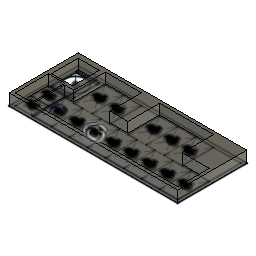
keyboard setup v5 (Autodesk Fusion 360 design; units mm, degrees)
Autodesk Fusion 360 part; units mm, degrees
sketch "Sketch1" plane through (0, 0, 0) normal (0, 0, 1) x (1, 0, 0)
  circle A0 centre (0, 0) radius 2
  line L0 (0, 0) -> (5.08, 0) construction
  circle A1 centre (5.08, 0) radius 0.85
  line L1 (0, 0) -> (2.54, 0) construction
  line L2 (2.54, 0) -> (2.54, 5.08) construction
  line L3 (2.54, 5.08) -> (0, 5.08) construction
  line L4 (0, 5.08) -> (0, 0) construction
  circle A2 centre (2.54, 5.08) radius 1.25
  line L5 (0, 0) -> (-3.81, 0) construction
  line L6 (-3.81, 0) -> (-3.81, 2.54) construction
  line L7 (-3.81, 2.54) -> (0, 2.54) construction
  line L8 (0, 2.54) -> (0, 0) construction
  circle A3 centre (-3.81, 2.54) radius 1.25
  circle A4 centre (-5.08, 0) radius 0.85
  line L9 (12, 21) -> (-12, 21)
  line L10 (-12, 21) -> (-12, -21)
  line L11 (-12, -21) -> (12, -21)
  line L12 (12, -21) -> (12, 21) construction
  line L13 (12, 21) -> (-12, -21) construction
  line L14 (-12, 21) -> (12, -21) construction
  line L15 (12, 21) -> (12, -21) construction
  line L16 (36, 21) -> (12, 21) construction
  line L17 (12, -21) -> (36, -21)
  line L18 (26.54, 5.08) -> (24, 5.08) construction
  line L19 (36, 21) -> (12, -21) construction
  line L20 (12, 21) -> (36, -21) construction
  circle A5 centre (24, 0) radius 2
  line L21 (36, -21) -> (36, 21) construction
  line L22 (24, 5.08) -> (24, 0) construction
  line L23 (24, 0) -> (29.08, 0) construction
  circle A6 centre (20.19, 2.54) radius 1.25
  line L24 (24, 2.54) -> (24, 0) construction
  line L25 (24, 0) -> (26.54, 0) construction
  circle A7 centre (18.92, 0) radius 0.85
  circle A8 centre (29.08, 0) radius 0.85
  line L26 (24, 0) -> (20.19, 0) construction
  line L27 (26.54, 0) -> (26.54, 5.08) construction
  circle A9 centre (26.54, 5.08) radius 1.25
  line L28 (20.19, 0) -> (20.19, 2.54) construction
  line L29 (20.19, 2.54) -> (24, 2.54) construction
  line L30 (36, 21) -> (36, -21) construction
  line L31 (60, 21) -> (36, 21)
  line L32 (36, -21) -> (60, -21)
  line L33 (50.54, 5.08) -> (48, 5.08) construction
  line L34 (60, 21) -> (36, -21) construction
  line L35 (36, 21) -> (60, -21) construction
  circle A10 centre (48, 0) radius 2
  line L36 (60, -21) -> (60, 21) construction
  line L37 (48, 5.08) -> (48, 0) construction
  line L38 (48, 0) -> (53.08, 0) construction
  circle A11 centre (44.19, 2.54) radius 1.25
  line L39 (48, 2.54) -> (48, 0) construction
  line L40 (48, 0) -> (50.54, 0) construction
  circle A12 centre (42.92, 0) radius 0.85
  circle A13 centre (53.08, 0) radius 0.85
  line L41 (48, 0) -> (44.19, 0) construction
  line L42 (50.54, 0) -> (50.54, 5.08) construction
  circle A14 centre (50.54, 5.08) radius 1.25
  line L43 (44.19, 0) -> (44.19, 2.54) construction
  line L44 (44.19, 2.54) -> (48, 2.54) construction
  line L45 (60, 21) -> (60, -21) construction
  line L46 (84, 21) -> (60, 21)
  line L47 (60, -21) -> (84, -21)
  line L48 (74.54, 5.08) -> (72, 5.08) construction
  line L49 (84, 21) -> (60, -21) construction
  line L50 (60, 21) -> (84, -21) construction
  circle A15 centre (72, 0) radius 2
  line L51 (84, -21) -> (84, 21) construction
  line L52 (72, 5.08) -> (72, 0) construction
  line L53 (72, 0) -> (77.08, 0) construction
  circle A16 centre (68.19, 2.54) radius 1.25
  line L54 (72, 2.54) -> (72, 0) construction
  line L55 (72, 0) -> (74.54, 0) construction
  circle A17 centre (66.92, 0) radius 0.85
  circle A18 centre (77.08, 0) radius 0.85
  line L56 (72, 0) -> (68.19, 0) construction
  line L57 (74.54, 0) -> (74.54, 5.08) construction
  circle A19 centre (74.54, 5.08) radius 1.25
  line L58 (68.19, 0) -> (68.19, 2.54) construction
  line L59 (68.19, 2.54) -> (72, 2.54) construction
  line L60 (84, 21) -> (84, -21) construction
  line L61 (108, 21) -> (84, 21) construction
  line L62 (84, -21) -> (108, -21)
  line L63 (98.54, 5.08) -> (96, 5.08) construction
  line L64 (108, 21) -> (84, -21) construction
  line L65 (84, 21) -> (108, -21) construction
  circle A20 centre (96, 0) radius 2
  line L66 (108, -21) -> (108, 21) construction
  line L67 (96, 5.08) -> (96, 0) construction
  line L68 (96, 0) -> (101.08, 0) construction
  circle A21 centre (92.19, 2.54) radius 1.25
  line L69 (96, 2.54) -> (96, 0) construction
  line L70 (96, 0) -> (98.54, 0) construction
  circle A22 centre (90.92, 0) radius 0.85
  circle A23 centre (101.08, 0) radius 0.85
  line L71 (96, 0) -> (92.19, 0) construction
  line L72 (98.54, 0) -> (98.54, 5.08) construction
  circle A24 centre (98.54, 5.08) radius 1.25
  line L73 (92.19, 0) -> (92.19, 2.54) construction
  line L74 (92.19, 2.54) -> (96, 2.54) construction
  line L75 (108, 21) -> (108, -21) construction
  line L76 (132, 21) -> (108, 21) construction
  line L77 (108, -21) -> (132, -21)
  line L78 (122.54, 5.08) -> (120, 5.08) construction
  line L79 (132, 21) -> (108, -21) construction
  line L80 (108, 21) -> (132, -21) construction
  circle A25 centre (120, 0) radius 2
  line L81 (132, -21) -> (132, 21) construction
  line L82 (120, 5.08) -> (120, 0) construction
  line L83 (120, 0) -> (125.08, 0) construction
  circle A26 centre (116.19, 2.54) radius 1.25
  line L84 (120, 2.54) -> (120, 0) construction
  line L85 (120, 0) -> (122.54, 0) construction
  circle A27 centre (114.92, 0) radius 0.85
  circle A28 centre (125.08, 0) radius 0.85
  line L86 (120, 0) -> (116.19, 0) construction
  line L87 (122.54, 0) -> (122.54, 5.08) construction
  circle A29 centre (122.54, 5.08) radius 1.25
  line L88 (116.19, 0) -> (116.19, 2.54) construction
  line L89 (116.19, 2.54) -> (120, 2.54) construction
  line L90 (132, 21) -> (132, -21) construction
  line L91 (156, 21) -> (132, 21)
  line L92 (132, -21) -> (156, -21)
  line L93 (146.54, 5.08) -> (144, 5.08) construction
  line L94 (156, 21) -> (132, -21) construction
  line L95 (132, 21) -> (156, -21) construction
  circle A30 centre (144, 0) radius 2
  line L96 (156, -21) -> (156, 21) construction
  line L97 (144, 5.08) -> (144, 0) construction
  line L98 (144, 0) -> (149.08, 0) construction
  circle A31 centre (140.19, 2.54) radius 1.25
  line L99 (144, 2.54) -> (144, 0) construction
  line L100 (144, 0) -> (146.54, 0) construction
  circle A32 centre (138.92, 0) radius 0.85
  circle A33 centre (149.08, 0) radius 0.85
  line L101 (144, 0) -> (140.19, 0) construction
  line L102 (146.54, 0) -> (146.54, 5.08) construction
  circle A34 centre (146.54, 5.08) radius 1.25
  line L103 (140.19, 0) -> (140.19, 2.54) construction
  line L104 (140.19, 2.54) -> (144, 2.54) construction
  line L105 (156, 21) -> (156, -21) construction
  line L106 (180, 21) -> (156, 21)
  line L107 (156, -21) -> (180, -21)
  line L108 (170.54, 5.08) -> (168, 5.08) construction
  line L109 (180, 21) -> (156, -21) construction
  line L110 (156, 21) -> (180, -21) construction
  circle A35 centre (168, 0) radius 2
  line L111 (180, -21) -> (180, 21)
  line L112 (168, 5.08) -> (168, 0) construction
  line L113 (168, 0) -> (173.08, 0) construction
  circle A36 centre (164.19, 2.54) radius 1.25
  line L114 (168, 2.54) -> (168, 0) construction
  line L115 (168, 0) -> (170.54, 0) construction
  circle A37 centre (162.92, 0) radius 0.85
  circle A38 centre (173.08, 0) radius 0.85
  line L116 (168, 0) -> (164.19, 0) construction
  line L117 (170.54, 0) -> (170.54, 5.08) construction
  circle A39 centre (170.54, 5.08) radius 1.25
  line L118 (164.19, 0) -> (164.19, 2.54) construction
  line L119 (164.19, 2.54) -> (168, 2.54) construction
  line L120 (48, 0) -> (53.08, 0) construction
  circle A40 centre (48, 0) radius 2
  line L121 (50.54, 5.08) -> (48, 5.08) construction
  circle A41 centre (42.92, 0) radius 0.85
  line L122 (48, 0) -> (44.19, 0) construction
  line L123 (44.19, 2.54) -> (48, 2.54) construction
  circle A42 centre (50.54, 5.08) radius 0.75
  circle A43 centre (53.08, 0) radius 0.85
  line L124 (50.54, 0) -> (50.54, 5.08) construction
  circle A44 centre (44.19, 2.54) radius 0.75
  line L125 (48, 5.08) -> (48, 0) construction
  line L126 (44.19, 0) -> (44.19, 2.54) construction
  line L127 (48, 2.54) -> (48, 0) construction
  line L128 (48, 0) -> (50.54, 0) construction
  line L129 (8.19, 44.54) -> (12, 44.54) construction
  circle A45 centre (6.92, 42) radius 0.85
  line L130 (12, 42) -> (8.19, 42) construction
  line L131 (12, 44.54) -> (12, 42) construction
  circle A46 centre (17.08, 42) radius 0.85
  line L132 (14.54, 42) -> (14.54, 47.08) construction
  circle A47 centre (12, 42) radius 2
  line L133 (14.54, 47.08) -> (12, 47.08) construction
  circle A48 centre (14.54, 47.08) radius 1.25
  circle A49 centre (8.19, 44.54) radius 1.25
  line L134 (12, 42) -> (14.54, 42) construction
  line L135 (12, 42) -> (17.08, 42) construction
  line L136 (12, 47.08) -> (12, 42) construction
  line L137 (8.19, 42) -> (8.19, 44.54) construction
  line L138 (24, 63) -> (0, 63) construction
  line L139 (0, 63) -> (0, 21)
  line L140 (0, 21) -> (24, 21) construction
  line L141 (24, 21) -> (24, 63) construction
  line L142 (24, 63) -> (0, 21) construction
  line L143 (0, 63) -> (24, 21) construction
  circle A50 centre (36, 42) radius 2
  line L144 (32.19, 44.54) -> (36, 44.54) construction
  line L145 (36, 42) -> (41.08, 42) construction
  line L146 (48, 63) -> (24, 63) construction
  circle A51 centre (38.54, 47.08) radius 1.25
  line L147 (24, 63) -> (24, 21) construction
  line L148 (24, 21) -> (48, 21) construction
  line L149 (48, 63) -> (24, 21) construction
  circle A52 centre (30.92, 42) radius 0.85
  line L150 (36, 47.08) -> (36, 42) construction
  line L151 (36, 42) -> (32.19, 42) construction
  line L152 (36, 42) -> (38.54, 42) construction
  line L153 (36, 44.54) -> (36, 42) construction
  circle A53 centre (41.08, 42) radius 0.85
  line L154 (32.19, 42) -> (32.19, 44.54) construction
  circle A54 centre (32.19, 44.54) radius 1.25
  line L155 (38.54, 47.08) -> (36, 47.08) construction
  line L156 (38.54, 42) -> (38.54, 47.08) construction
  line L157 (24, 63) -> (48, 21) construction
  line L158 (48, 21) -> (48, 63)
  line L159 (96, 63) -> (72, 63) construction
  line L160 (84, 44.54) -> (84, 42) construction
  circle A55 centre (102.92, 42) radius 0.85
  line L161 (108, 42) -> (104.19, 42) construction
  line L162 (104.19, 42) -> (104.19, 44.54) construction
  circle A56 centre (86.54, 47.08) radius 1.25
  line L163 (84, 42) -> (86.54, 42) construction
  line L164 (84, 47.08) -> (84, 42) construction
  circle A57 centre (110.54, 47.08) radius 1.25
  circle A58 centre (80.19, 44.54) radius 1.25
  line L165 (84, 42) -> (80.19, 42) construction
  line L166 (108, 47.08) -> (108, 42) construction
  line L167 (96, 21) -> (96, 63) construction
  line L168 (120, 63) -> (96, 21) construction
  circle A59 centre (113.08, 42) radius 0.85
  circle A60 centre (108, 42) radius 2
  line L169 (120, 63) -> (96, 63) construction
  line L170 (110.54, 47.08) -> (108, 47.08) construction
  line L171 (86.54, 47.08) -> (84, 47.08) construction
  line L172 (96, 21) -> (120, 21) construction
  line L173 (86.54, 42) -> (86.54, 47.08) construction
  line L174 (96, 63) -> (120, 21) construction
  line L175 (108, 44.54) -> (108, 42) construction
  circle A61 centre (84, 42) radius 2
  circle A62 centre (78.92, 42) radius 0.85
  line L176 (108, 42) -> (110.54, 42) construction
  line L177 (80.19, 44.54) -> (84, 44.54) construction
  line L178 (72, 21) -> (96, 21) construction
  line L179 (104.19, 44.54) -> (108, 44.54) construction
  circle A63 centre (104.19, 44.54) radius 1.25
  line L180 (120, 21) -> (120, 63) construction
  line L181 (80.19, 42) -> (80.19, 44.54) construction
  line L182 (72, 63) -> (96, 21) construction
  line L183 (84, 42) -> (89.08, 42) construction
  line L184 (110.54, 42) -> (110.54, 47.08) construction
  line L185 (96, 63) -> (72, 21) construction
  circle A64 centre (89.08, 42) radius 0.85
  line L186 (108, 42) -> (113.08, 42) construction
  line L187 (72, 63) -> (72, 21)
  line L188 (96, 63) -> (96, 21) construction
  circle A65 centre (132, 42) radius 2
  line L189 (128.19, 44.54) -> (132, 44.54) construction
  line L190 (132, 42) -> (137.08, 42) construction
  line L191 (144, 63) -> (120, 63) construction
  circle A66 centre (134.54, 47.08) radius 1.25
  line L192 (120, 63) -> (120, 21) construction
  line L193 (120, 21) -> (144, 21) construction
  line L194 (144, 63) -> (120, 21) construction
  circle A67 centre (126.92, 42) radius 0.85
  line L195 (132, 47.08) -> (132, 42) construction
  line L196 (132, 42) -> (128.19, 42) construction
  line L197 (132, 42) -> (134.54, 42) construction
  line L198 (132, 44.54) -> (132, 42) construction
  circle A68 centre (137.08, 42) radius 0.85
  line L199 (128.19, 42) -> (128.19, 44.54) construction
  circle A69 centre (128.19, 44.54) radius 1.25
  line L200 (134.54, 47.08) -> (132, 47.08) construction
  line L201 (134.54, 42) -> (134.54, 47.08) construction
  line L202 (120, 63) -> (144, 21) construction
  line L203 (144, 21) -> (144, 63)
  line L204 (-12, -21) -> (180, -21)
  line L205 (180, -21) -> (180, 63)
  line L206 (180, 63) -> (-12, 63)
  line L207 (-12, 63) -> (-12, -21)
  circle A70 centre (-25, -10) radius 2
  line L208 (-25, -7.46) -> (-25, -10) construction
  circle A71 centre (-22.46, -4.92) radius 1.25
  line L209 (-25, -4.92) -> (-25, -10) construction
  circle A72 centre (-30.08, -10) radius 0.85
  line L210 (-28.81, -7.46) -> (-25, -7.46) construction
  line L211 (-25, -10) -> (-22.46, -10) construction
  circle A73 centre (-19.92, -10) radius 0.85
  line L212 (-25, -10) -> (-28.81, -10) construction
  line L213 (-22.46, -10) -> (-22.46, -4.92) construction
  line L214 (-22.46, -4.92) -> (-25, -4.92) construction
  circle A74 centre (-28.81, -7.46) radius 1.25
  line L215 (-28.81, -10) -> (-28.81, -7.46) construction
  line L216 (-25, -10) -> (-19.92, -10) construction
  line L217 (-14, 1) -> (-36, 1)
  line L218 (-36, 1) -> (-36, -21)
  line L219 (-36, -21) -> (-14, -21)
  line L220 (-14, -21) -> (-14, 1)
  line L221 (-14, 1) -> (-36, -21) construction
  line L222 (-36, 1) -> (-14, -21) construction
  line L223 (-36, 23) -> (-14, 1) construction
  line L224 (-25, 12) -> (-22.46, 12) construction
  line L225 (-28.81, 12) -> (-28.81, 14.54) construction
  line L226 (-28.81, 14.54) -> (-25, 14.54) construction
  line L227 (-36, 23) -> (-36, 1)
  line L228 (-36, 1) -> (-14, 1)
  line L229 (-25, 12) -> (-19.92, 12) construction
  line L230 (-25, 14.54) -> (-25, 12) construction
  circle A75 centre (-19.92, 12) radius 0.85
  line L231 (-14, 23) -> (-36, 23)
  line L232 (-25, 12) -> (-28.81, 12) construction
  line L233 (-25, 17.08) -> (-25, 12) construction
  circle A76 centre (-22.46, 17.08) radius 1.25
  circle A77 centre (-28.81, 14.54) radius 1.25
  line L234 (-14, 23) -> (-36, 1) construction
  line L235 (-14, 1) -> (-14, 23)
  circle A78 centre (-30.08, 12) radius 0.85
  line L236 (-22.46, 17.08) -> (-25, 17.08) construction
  line L237 (-22.46, 12) -> (-22.46, 17.08) construction
  circle A79 centre (-25, 12) radius 2
  line L238 (-14, -21) -> (-12, -21)
  line L239 (-34, 25.25) -> (-6, 25.25)
  line L240 (-6, 25.25) -> (-6, 60.75)
  line L241 (-6, 60.75) -> (-34, 60.75)
  line L242 (-34, 60.75) -> (-34, 25.25)
  line L243 (-34, 60.75) -> (-6, 60.75)
  line L244 (-6, 60.75) -> (-6, 57.75)
  line L245 (-6, 57.75) -> (-34, 57.75)
  line L246 (-34, 57.75) -> (-34, 60.75)
  line L247 (-34, 25.25) -> (-6, 25.25)
  line L248 (-6, 25.25) -> (-6, 28.25)
  line L249 (-6, 28.25) -> (-34, 28.25)
  line L250 (-34, 28.25) -> (-34, 25.25)
  line L251 (-36, 23) -> (-12, 23)
  line L252 (-12, 23) -> (-12, 63)
  line L253 (-12, 63) -> (-36, 63)
  line L254 (-36, 63) -> (-36, 23)
  line L255 (-34, 57.75) -> (-6, 28.25) construction
  circle A80 centre (-20, 43) radius 14
  line L256 (-36, -21) -> (-40, -21) construction
  line L257 (-40, -21) -> (-40, -25) construction
  line L258 (-40, -25) -> (-36, -25) construction
  line L259 (-36, -25) -> (-36, -21) construction
  line L260 (180, 63) -> (184, 63) construction
  line L261 (184, 63) -> (184, 67) construction
  line L262 (184, 67) -> (180, 67) construction
  line L263 (180, 67) -> (180, 63) construction
  line L264 (184, 67) -> (-40, 67)
  line L265 (-40, 67) -> (-40, -25)
  line L266 (-40, -25) -> (184, -25)
  line L267 (184, -25) -> (184, 67)
  point P0 (24, 0)
  point P1 (24, 0)
  point P2 (48, 0)
  point P3 (48, 0)
  point P4 (72, 0)
  point P5 (72, 0)
  point P6 (96, 0)
  point P7 (96, 0)
  point P8 (120, 0)
  point P9 (120, 0)
  point P10 (144, 0)
  point P11 (144, 0)
  point P12 (168, 0)
  point P13 (168, 0)
  point P14 (48, 0)
  point P15 (48, 0)
  point P16 (12, 42)
  point P17 (12, 42)
  point P18 (12, 42)
  point P19 (36, 42)
  point P20 (36, 42)
  point P21 (36, 42)
  point P22 (108, 42)
  point P23 (108, 42)
  point P24 (108, 42)
  point P25 (84, 42)
  point P26 (84, 42)
  point P27 (84, 42)
  point P28 (132, 42)
  point P29 (132, 42)
  point P30 (132, 42)
  point P31 (-25, -10)
  point P32 (-25, -10)
  point P33 (-25, -10)
  point P34 (-25, 12)
  point P35 (-25, 12)
  point P36 (-25, 12)
  dimension "d1" = 4
  dimension "d2" = 5.08
  dimension "d3" = 1.7
  dimension "d4" = 2.54
  dimension "d5" = 5.08
  dimension "d6" = 2.5
  dimension "d7" = 3.81
  dimension "d8" = 2.54
  dimension "d9" = 2.5
  dimension "d10" = 24
  dimension "d11" = 42
  dimension "d16" = 24
  dimension "d17" = 0
  dimension "d18" = 4
  dimension "d19" = 5.08
  dimension "d20" = 1.7
  dimension "d21" = 2.54
  dimension "d22" = 5.08
  dimension "d23" = 2.5
  dimension "d24" = 3.81
  dimension "d25" = 2.54
  dimension "d26" = 2.5
  dimension "d27" = 24
  dimension "d28" = 42
  dimension "d31" = 24
  dimension "d32" = 0
  dimension "d35" = 48
  dimension "d36" = 0
  dimension "d37" = 4
  dimension "d38" = 5.08
  dimension "d39" = 1.7
  dimension "d40" = 2.54
  dimension "d41" = 5.08
  dimension "d42" = 2.5
  dimension "d43" = 3.81
  dimension "d44" = 2.54
  dimension "d45" = 2.5
  dimension "d46" = 24
  dimension "d47" = 42
  dimension "d48" = 4
  dimension "d49" = 5.08
  dimension "d50" = 1.7
  dimension "d51" = 2.54
  dimension "d52" = 5.08
  dimension "d53" = 2.5
  dimension "d54" = 3.81
  dimension "d55" = 2.54
  dimension "d56" = 2.5
  dimension "d57" = 22
  dimension "d58" = 22
  dimension "d61" = 0
  dimension "d62" = 22
  dimension "d63" = 2
  dimension "d64" = 28
  dimension "d65" = 35.5
  dimension "d66" = 3
  dimension "d67" = 3
  dimension "d68" = 2
  dimension "d69" = 2.25
  dimension "d72" = 4
  dimension "d73" = 4
  dimension "d74" = 4
  dimension "d75" = 4
  constraint coincident A0.centre L0.start
  constraint horizontal L0
  constraint coincident L0.end A1.centre
  constraint horizontal L1
  constraint vertical L2
  constraint horizontal L3
  constraint vertical L4
  constraint coincident L2.end L3.start
  constraint horizontal L5
  constraint vertical L6
  constraint horizontal L7
  constraint vertical L8
  constraint coincident L6.end L7.start
  constraint symmetric A1 L4 A4
  constraint horizontal L9
  constraint perpendicular L9 L10
  constraint parallel L9 L11
  constraint parallel L10 L12
  constraint coincident L13 A0.centre
  constraint coincident L14 A0.centre
  constraint coincident P18 P17
  constraint horizontal L135
  constraint coincident A46.centre L135.end
  constraint horizontal L134
  constraint vertical L132
  constraint horizontal L133
  constraint vertical L136
  constraint coincident L132.end L133.start
  constraint horizontal L130
  constraint vertical L137
  constraint horizontal L129
  constraint vertical L131
  constraint coincident L129.start A49.centre
  constraint symmetric A45 A46 L136
  constraint horizontal L138
  constraint perpendicular L138 L139
  constraint parallel L138 L140
  constraint parallel L139 L141
  constraint coincident L142 P18
  constraint coincident L143 P18
  constraint coincident P27 P26
  constraint horizontal L183
  constraint coincident L183.end A64.centre
  constraint horizontal L163
  constraint vertical L173
  constraint horizontal L171
  constraint vertical L164
  constraint coincident A56.centre L171.start
  constraint horizontal L165
  constraint vertical L181
  constraint horizontal L177
  constraint vertical L160
  constraint coincident A58.centre L177.start
  constraint symmetric L164 A62 A64
  constraint horizontal L159
  constraint perpendicular L159 L187
  constraint parallel L159 L178
  constraint parallel L167 L187
  constraint coincident P27 L185
  constraint coincident P27 L182
  constraint midpoint L31 L148.end
  constraint midpoint L91 L193.end
  constraint perpendicular L204 L205
  constraint parallel L204 L206
  constraint parallel L205 L207
  constraint coincident P33 P32
  constraint horizontal L216
  constraint coincident A73.centre L216.end
  constraint horizontal L211
  constraint vertical L213
  constraint horizontal L214
  constraint vertical L209
  constraint coincident A71.centre L213.end
  constraint horizontal L212
  constraint vertical L215
  constraint horizontal L210
  constraint vertical L208
  constraint coincident L210.start A74.centre
  constraint symmetric L209 A72 A73
  constraint horizontal L217
  constraint perpendicular L217 L218
  constraint parallel L217 L219
  constraint parallel L218 L220
  constraint coincident L221 P33
  constraint coincident L222 P33
  constraint horizontal L238
  constraint horizontal L239
  constraint vertical L240
  constraint horizontal L241
  constraint vertical L242
  constraint perpendicular L243 L244
  constraint parallel L243 L245
  constraint parallel L244 L246
  constraint perpendicular L247 L248
  constraint parallel L247 L249
  constraint parallel L248 L250
  constraint horizontal L251
  constraint vertical L252
  constraint horizontal L253
  constraint vertical L254
  constraint coincident L138.end L206
  constraint midpoint L255 A80.centre
  constraint tangent L242 A80
  constraint horizontal L256
  constraint vertical L257
  constraint horizontal L258
  constraint vertical L259
  constraint horizontal L260
  constraint vertical L261
  constraint horizontal L262
  constraint vertical L263
  constraint horizontal L264
  constraint vertical L265
  constraint horizontal L266
  constraint vertical L267
  measures "d1" diameter of A0
  measures "d2" distance of A0.centre L0.end
  measures "d3" diameter of A1
  measures "d4" distance of A0.centre L1.end
  measures "d5" distance of A0.centre L3.end
  measures "d6" diameter of A2
  measures "d7" distance of A0.centre L5.end
  measures "d8" distance of A0.centre L7.end
  measures "d9" diameter of A3
  measures "d10" distance of L10.end L11.end
  measures "d11" distance of L9.end L10.end
  measures "d18" diameter of A47
  measures "d19" distance of P18 A46.centre
  measures "d20" diameter of A46
  measures "d21" distance of P18 L132.start
  measures "d22" distance of P18 L133.end
  measures "d23" diameter of A48
  measures "d24" distance of P18 L130.end
  measures "d25" distance of P18 L129.end
  measures "d26" diameter of A49
  measures "d27" distance of L139.end L140.end
  measures "d28" distance of L138.end L139.end
  measures "d37" diameter of A61
  measures "d38" distance of P27 L183.end
  measures "d39" diameter of A64
  measures "d40" distance of L163.end P27
  measures "d41" distance of L164.start P27
  measures "d42" diameter of A56
  measures "d43" distance of P27 L165.end
  measures "d44" distance of L160.start P27
  measures "d45" diameter of A58
  measures "d46" distance of L178.start L167.start
  measures "d47" distance of L178.start L159.end
  measures "d48" diameter of A70
  measures "d49" distance of P33 A73.centre
  measures "d50" diameter of A73
  measures "d51" distance of P33 L211.end
  measures "d52" distance of P33 L209.start
  measures "d53" diameter of A71
  measures "d54" distance of P33 L212.end
  measures "d55" distance of P33 L208.start
  measures "d56" diameter of A74
  measures "d57" distance of L218.end L219.end
  measures "d58" distance of L217.end L218.end
  measures "d63" distance of L10 L220
  measures "d64" distance of L239.start L239.end
  measures "d65" distance of L239.start L241.end
  measures "d66" distance of L241.end L245.end
  measures "d67" distance of L239.start L249.end
  measures "d68" distance of L242 L254
  measures "d69" distance of L241 L253
  measures "d72" distance of L218.end L256.end
  measures "d73" distance of L218.end L258.end
  measures "d74" distance of L205.end L260.end
  measures "d75" distance of L205.end L262.end
extrude "Extrude1" add sketch "Sketch1" along normal blind 1.5 contours L9 L10 L11 L17 L31 L32 L46 L47 L62 L77 L91 L92 L106 L107 L111 L139 L158 L187 L203 L204 L205 L206 L207 | L217 L218 L219 L220 L228 | L207 L239 L242 L247 L249 L250 L252 | L207 L239 L240 L247 L248 L249 L252 | L217 L227 L228 L231 L235 L251 | L207 L240 L241 L243 L244 L245 L252 | L207 L241 L242 L243 L245 L246 L252 makes body 1 at (80.0697, -14.663, 0) makes body 2 at (-24.9502, -17.9981, 1.5) makes body 3 at (-24.6667, 59.75, 0) makes body 4 at (-24.6667, 27.25, 0)
extrude "Extrude3" add sketch "Sketch1" along normal blind 15 contours L9 L139 L206 L207 L239 L240 L241 L243 L244 L247 L248 L252 | L10 L207 L220 L235 L238 L251 | L207 L231 L239 L241 L242 L243 L246 L247 L250 L251 L252 L253 L254 | L31 L46 L158 L187 L206 | L91 L106 L203 L205 L206 | L264 L265 L266 L267 bodies 1 2
equation "d2 = ( 4 * 1.27 ) * 1 mm"
equation "d4 = ( 2 * 1.27 ) * 1 mm"
equation "d5 = ( 4 * 1.27 ) * 1 mm"
equation "d7 = ( 3 * 1.27 ) * 1 mm"
equation "d8 = ( 2 * 1.27 ) * 1 mm"
equation "d19 = ( 4 * 1.27 ) * 1 mm"
equation "d21 = ( 2 * 1.27 ) * 1 mm"
equation "d22 = ( 4 * 1.27 ) * 1 mm"
equation "d24 = ( 3 * 1.27 ) * 1 mm"
equation "d25 = ( 2 * 1.27 ) * 1 mm"
equation "d38 = ( 4 * 1.27 ) * 1 mm"
equation "d40 = ( 2 * 1.27 ) * 1 mm"
equation "d41 = ( 4 * 1.27 ) * 1 mm"
equation "d43 = ( 3 * 1.27 ) * 1 mm"
equation "d44 = ( 2 * 1.27 ) * 1 mm"
equation "d49 = ( 4 * 1.27 ) * 1 mm"
equation "d51 = ( 2 * 1.27 ) * 1 mm"
equation "d52 = ( 4 * 1.27 ) * 1 mm"
equation "d54 = ( 3 * 1.27 ) * 1 mm"
equation "d55 = ( 2 * 1.27 ) * 1 mm"
